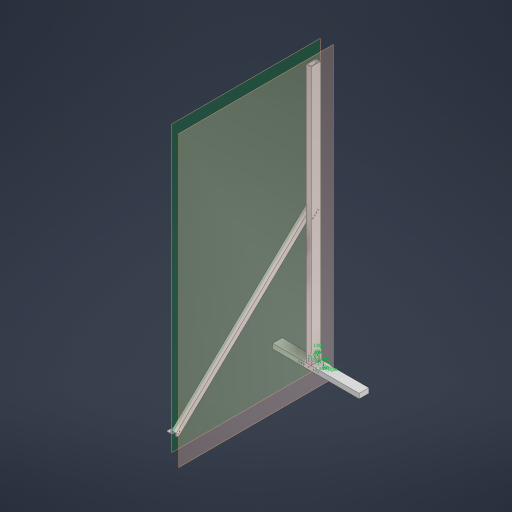
# Autodesk Inventor part: Truss
Saved by Autodesk Inventor 2023 (Build 270158000, 158)
## iProperties
Created: 2023-01-10
Part Number: Truss
Material: Generic
Document SubType Name: Modeling
Designer: Terrence
Density: 1 g/cm^3
Appearance: Default
Author: Terrence
Autodesk Inventor part; units mm, degrees
ref_plane "YZ Plane" through (0, 0, 0) normal (1, 0, 0) x (0, 1, 0)
ref_plane "XZ Plane" through (0, 0, 0) normal (0, 1, 0) x (-1, 0, 0)
ref_plane "XY Plane" through (0, 0, 0) normal (0, 0, 1) x (1, 0, 0)
sketch "Sketch1" plane through (0, 0, 0) normal (0, 1, 0) x (-1, 0, 0)
  line L0 (0, 0) -> (-25.4, 0)
  line L1 (-25.4, 0) -> (-25.4, -50.8)
  line L2 (-25.4, -50.8) -> (0, -50.8)
  line L3 (0, -50.8) -> (0, 0)
  dimension "d0" = 25.4
  dimension "d1" = 50.8
  constraints: 8 end point, 2 parallel, 1 horizontal, 1 perpendicular
  measures "d0" distance of L2.end L1.end
  measures "d1" distance of L1.end L0.end
extrude "Extrusion1" add sketch "Sketch1" along normal blind 1365.885
shell "Shell1" thickness 3.175 removed faces 2 at (16.9333, 1365.885, -33.8667) at (16.9333, 0, -33.8667)
sketch "Sketch12" plane through (0, 0, -50.8) normal (-1, 0, 0) x (0, 0, 1)
  line L0 (3.175, 1365.885) -> (47.625, 1365.885) projected
  line L1 (50.8, 0) -> (50.8, 1365.885) projected
  line L2 (0, 0) -> (0, 1365.885) projected
  line L3 (25.4, 0) -> (711.962, 0)
  line L4 (47.625, 0) -> (3.175, 0) projected
  line L5 (711.962, 0) -> (711.962, 3.429)
  line L6 (711.962, 3.429) -> (454.4895, 3.429)
  line L7 (8.7645, 698.8061) -> (700.8631, 38.8235) construction
  line L8 (711.962, 3.429) -> (737.362, 3.429) construction
  line L9 (737.362, 3.429) -> (737.362, 28.829) construction
  line L10 (737.362, 28.829) -> (711.962, 28.829) construction
  line L11 (711.962, 28.829) -> (711.962, 3.429) construction
  line L12 (0, 689.6151) -> (719.5773, 3.429)
  line L13 (692.0986, 29.6325) -> (709.6276, 48.0145) construction
  line L14 (709.6276, 48.0145) -> (737.362, 21.5671) construction
  line L15 (17.529, 707.997) -> (0, 689.6151)
  line L16 (0, 689.6151) -> (709.6276, 48.0145) construction
  line L17 (692.0986, 29.6325) -> (17.529, 707.997) construction
  line L18 (711.962, 28.829) -> (737.362, 3.429) construction
  line L19 (737.362, 21.5671) -> (17.529, 707.997)
  line L20 (719.5773, 3.429) -> (692.0986, 29.6325) construction
  line L21 (737.362, 21.5671) -> (737.362, 3.429)
  line L22 (719.5773, 3.429) -> (737.362, 3.429)
  line L23 (25.4, 0) -> (25.4, 0)
  line L24 (25.4, 0) -> (25.4, 1365.885) construction
  point P0 (354.8138, 368.8148)
  point P1 (724.662, 16.129)
  point P2 (747.538, -137.3809)
  point P3 (729.3381, -137.3809)
  point P4 (25.4, 682.9425)
  dimension "d84" = 686.562
  dimension "d85" = 3.429
  dimension "d86" = 25.4
  dimension "d87" = 25.4
  dimension "d88" = 25.4
  dimension "d112" = 0
  constraints: 42 end point, 8 midpoint, 7 parallel, 5 perpendicular, 4 point on line, 3 vertical, 1 collinear, 1 horizontal, 2 other
  measures "d84" distance of L3.start L3.end
  measures "d85" distance of L3.end L5.end
  measures "d86" distance of L10.end L9.end
  measures "d87" distance of L9.end L8.end
  measures "d88" distance of L13.start L13.end
  measures "d112" distance of L23.start L3.start
extrude "Extrusion9" add sketch "Sketch12" along normal blind 25.4 separate body
sketch "Sketch17" plane through (-25.4, 0, -50.8) normal (-1, 0, 0) x (0, 0, 1)
  line L0 (25.4, 0) -> (711.962, 0) projected
  line L1 (711.962, 0) -> (711.962, 3.429) projected
  line L2 (711.962, 3.429) -> (754.4394, 3.429) construction
  line L3 (711.962, 3.429) -> (737.362, 3.429)
  line L4 (737.362, 3.429) -> (737.362, 28.829)
  line L5 (737.362, 28.829) -> (711.962, 28.829)
  line L6 (711.962, 28.829) -> (711.962, 3.429)
  point P0 (50.8, 0)
  dimension "d89" = 25.4
  dimension "d90" = 25.4
  constraints: 10 end point, 2 horizontal, 2 parallel, 1 perpendicular
  measures "d89" distance of L5.end L4.end
  measures "d90" distance of L4.end L3.end
extrude "Extrusion13" add sketch "Sketch17" along normal blind 3.175 separate body
sketch "Sketch18" plane through (-28.575, 0, -50.8) normal (-1, 0, 0) x (0, 0, 1)
  line L0 (711.962, 28.829) -> (711.962, 3.429) projected
  line L1 (711.962, 3.429) -> (737.362, 3.429)
  line L2 (737.362, 3.429) -> (737.362, 6.604)
  line L3 (737.362, 6.604) -> (711.962, 6.604)
  line L4 (711.962, 6.604) -> (711.962, 3.429)
  point P0 (50.8, 0)
  dimension "d93" = 25.4
  dimension "d94" = 3.175
  constraints: 8 end point, 2 parallel, 1 horizontal, 1 perpendicular
  measures "d93" distance of L3.end L2.end
  measures "d94" distance of L2.end L1.end
extrude "Extrusion14" add sketch "Sketch18" along normal blind 21.7714 bodies 3
shell "Shell4" thickness 3.175 removed faces 3 at (-8.4667, 701.8697, -39.114) at (-16.9333, 9.475, 686.562) at (-16.9333, 3.429, 674.7055) bodies 2
sketch "Sketch20" plane through (-28.575, 0, -50.8) normal (-1, 0, 0) x (0, 0, 1)
  line L0 (737.362, 28.829) -> (711.962, 28.829) projected
  line L1 (737.362, 3.429) -> (737.362, 28.829) projected
  line L2 (711.962, 28.829) -> (737.362, 3.429) construction
  circle A0 centre (720.9423, 19.8487) radius 2.667
  circle A1 centre (728.3817, 12.4093) radius 2.667
  point P0 (50.8, 0)
  point P1 (724.662, 16.129)
  dimension "d105" = 5.334
  dimension "d106" = 5.334
  dimension "d110" = 12.7
  dimension "d111" = 12.7
  constraints: 2 centre point, 2 end point, 2 point on line, 1 midpoint
  measures "d105" diameter of A0
  measures "d106" diameter of A1
  measures "d110" distance of L0.end A0.centre
  measures "d111" distance of L1.start A1.centre
extrude "Extrusion16" cut sketch "Sketch20" against normal through all bodies 3 2
sketch "Sketch19" plane through (-25.4, 0, -50.8) normal (-1, 0, 0) x (0, 0, 1)
  line L0 (17.529, 707.997) -> (0, 689.6151) projected
  line L1 (8.7645, 698.8061) -> (708.4549, 31.584) construction
  circle A0 centre (13.36, 694.4238) radius 2.667
  circle A1 centre (22.5509, 685.6594) radius 2.667
  circle A2 centre (31.7419, 676.8949) radius 2.667
  circle A3 centre (40.9329, 668.1304) radius 2.667
  point P0 (50.8, 0)
  dimension "d97" = 5.334
  dimension "d98" = 6.35
  dimension "d99" = 12.7
  dimension "d100" = 12.7
  dimension "d101" = 12.7
  constraints: 4 centre point, 4 point on line, 3 equal radius, 2 end point, 1 midpoint, 1 perpendicular
  measures "d97" diameter of A0
  measures "d98" distance from line of L0 A0.centre
  measures "d99" distance of A1.centre A0.centre
  measures "d100" distance of A2.centre A1.centre
  measures "d101" distance of A3.centre A2.centre
extrude "Extrusion15" cut sketch "Sketch19" against normal through all bodies 1 2
ref_plane "Work Plane3" through (-12.7, 0, -50.8) normal (-1, 0, 0) x (0, 0, 1)
sketch "Sketch21" plane through (0, 0, -50.8) normal (0, 0, -1) x (-1, 0, 0)
  line L0 (0, -25.4) -> (-25.4, -25.4)
  line L1 (-25.4, -25.4) -> (-25.4, 50.8)
  line L2 (-25.4, 50.8) -> (0, 50.8)
  line L3 (0, 50.8) -> (0, -25.4)
  line L4 (0, -25.4) -> (-76.2, -25.4)
  line L5 (-76.2, -25.4) -> (-76.2, 0)
  line L6 (-76.2, 0) -> (0, 0)
  line L7 (0, 0) -> (0, -25.4)
  line L8 (-12.7, 50.8) -> (-12.7, -25.4) construction
  line L9 (-76.2, -12.7) -> (0, -12.7) construction
  circle A0 centre (-12.7, -12.7) radius 2.667
  circle A1 centre (-12.7, 12.7) radius 2.667
  circle A2 centre (-12.7, 25.4) radius 2.667
  circle A3 centre (-12.7, 38.1) radius 2.667
  circle A4 centre (-38.1, -12.7) radius 2.667
  circle A5 centre (-50.8, -12.7) radius 2.667
  circle A6 centre (-63.5, -12.7) radius 2.667
  line L10 (-25.4, -25.4) -> (50.8, -25.4)
  line L11 (50.8, -25.4) -> (50.8, 0)
  line L12 (50.8, 0) -> (-25.4, 0)
  circle A7 centre (12.7, -12.7) radius 2.667
  circle A8 centre (25.4, -12.7) radius 2.667
  circle A9 centre (38.1, -12.7) radius 2.667
  point P0 (-38.1, -12.7)
  point P1 (-12.7, 12.7)
  point P2 (-25.4, 0)
  dimension "d139" = 25.4
  dimension "d140" = 76.2
  dimension "d141" = 76.2
  dimension "d142" = 25.4
  dimension "d143" = 25.4
  dimension "d144" = 25.4
  dimension "d145" = 5.334
  dimension "d146" = 12.7
  dimension "d147" = 12.7
  dimension "d148" = 12.7
  dimension "d149" = 12.7
  constraints: 26 end point, 10 centre point, 7 midpoint, 7 point on line, 6 equal radius, 6 symmetric about line, 4 parallel, 3 perpendicular, 2 horizontal, 1 coincident, 3 other
  measures "d139" distance of L1.end L2.end
  measures "d140" distance of L0.end L1.end
  measures "d141" distance of L5.end L6.end
  measures "d142" distance of L4.end L5.end
  measures "d143" distance of A0.centre A4.centre
  measures "d144" distance of A1.centre A0.centre
  measures "d145" diameter of A0
  measures "d146" distance of point (-38.1, -12.7) A5.centre
  measures "d147" distance of A5.centre A6.centre
  measures "d148" distance of A2.centre point (-12.7, 12.7)
  measures "d149" distance of A2.centre A3.centre
sketch "Sketch22" plane through (25.4, 0, 0) normal (1, 0, 0) x (0, 0, -1)
  line L0 (0, -25.4) -> (50.8, -25.4)
  line L1 (50.8, -25.4) -> (50.8, 0)
  line L2 (50.8, 0) -> (0, 0)
  line L3 (0, 0) -> (0, -25.4)
  dimension "d133" = 50.8
  dimension "d134" = 25.4
  constraints: 8 end point, 2 parallel, 1 coincident, 1 horizontal, 1 perpendicular
  measures "d133" distance of L2.end L1.end
  measures "d134" distance of L1.end L0.end
extrude "Extrusion18" add sketch "Sketch22" along normal blind 254 and the other way blind 203.2 separate body
extrude "Extrusion19" add sketch "Sketch21" along normal blind 3.175 separate body
ref_plane "Work Plane4" through (50.8, 0, 0) normal (1, 0, 0) x (0, 0, -1)
extrude "Extrusion20" cut sketch "Sketch21" against normal through all contours A0 | A1 | A2 | A3 | A4 | A5 | A6 | A7 | A8 | A9 bodies 1 4
body "Solid1"
body "Solid6"
body "Solid7"
body "Solid10"
body "Solid12"
